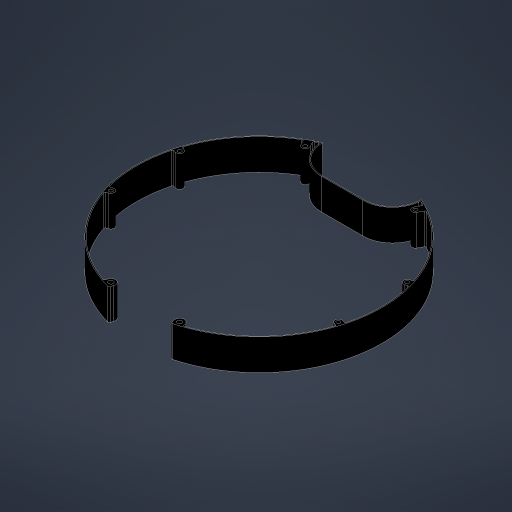
# Autodesk Inventor part: Schutz4
Saved by Autodesk Inventor 2023 (Build 270158000, 158)
## iProperties
Created: 2023-02-26
Part Number: Schutz4
Material: Generic
Document SubType Name: Modeling
Designer: Elias Braun
Density: 1 g/cm^3
Appearance: Default
Author: Elias Braun
Autodesk Inventor part; units mm, degrees
ref_plane "YZ Plane" through (0, 0, 0) normal (1, 0, 0) x (0, 1, 0)
ref_plane "XZ Plane" through (0, 0, 0) normal (0, 1, 0) x (-1, 0, 0)
ref_plane "XY Plane" through (0, 0, 0) normal (0, 0, 1) x (1, 0, 0)
sketch "Sketch1" plane through (0, 0, 0) normal (0, 1, 0) x (-1, 0, 0)
  circle A0 centre (0, 0) radius 103.75 construction
  line L0 (0, -103.75) -> (-30, -103.75) construction
  line L1 (-30, -103.75) -> (-30, -99.318) construction
  line L2 (0, -103.75) -> (0, -91.6543) construction
  line L3 (0, 0) -> (-10.2863, 0) construction
  circle A1 centre (-30, -99.318) radius 1.6
  circle A2 centre (30, -99.318) radius 1.6
  circle A3 centre (-99.318, -30) radius 1.6
  circle A4 centre (-99.318, 30) radius 1.6
  arc A5 (53.1423, -96.3114) -> (51.7739, -97.0539) centre (0, 0) ccw construction
  arc A6 (43.0581, -98.5) -> (-43.0581, -98.5) centre (0, 0) ccw
  line L4 (0, -107.5) -> (0, -98.5) construction
  line L5 (0, -98.5) -> (0, -73.5) construction
  line L6 (0, -98.5) -> (-43.0581, -98.5) construction
  line L7 (0, -98.5) -> (43.0581, -98.5) construction
  line L8 (43.0581, -98.5) -> (-43.0581, -98.5) construction
  line L9 (-18.0581, -73.5) -> (18.0581, -73.5)
  arc A7 (43.0581, -98.5) -> (18.0581, -73.5) centre (18.0581, -98.5) ccw
  arc A8 (-18.0581, -73.5) -> (-43.0581, -98.5) centre (-18.0581, -98.5) ccw
  line L10 (0, 107.5) -> (0, 97.5) construction
  line L11 (0, 97.5) -> (-22.5, 97.5) construction
  line L12 (-22.5, 97.5) -> (-22.5, 82.5) construction
  line L13 (22.5, 82.5) -> (22.5, 97.5) construction
  line L14 (22.5, 90) -> (-22.5, 90) construction
  line L15 (15, 97.5) -> (-15, 97.5)
  line L16 (-15, 82.5) -> (15, 82.5)
  arc A9 (15, 82.5) -> (15, 97.5) centre (15, 90) ccw
  arc A10 (-15, 97.5) -> (-15, 82.5) centre (-15, 90) ccw
  line L17 (22.5, 82.5) -> (17.5, 82.5) construction
  line L18 (17.5, 82.5) -> (17.5, 77.5) construction
  circle A11 centre (17.5, 77.5) radius 1.6
  circle A12 centre (-17.5, 77.5) radius 1.6
  line L19 (-58.3363, 79.5495) -> (-79.5495, 58.3363)
  arc A13 (-47.7297, 68.9429) -> (-58.3363, 79.5495) centre (-53.033, 74.2462) ccw
  arc A14 (-79.5495, 58.3363) -> (-68.9429, 47.7297) centre (-74.2462, 53.033) ccw
  line L20 (-68.9429, 47.7297) -> (-47.7297, 68.9429)
  circle A15 centre (-67.1751, 42.4264) radius 1.6
  circle A16 centre (-42.4264, 67.1751) radius 1.6
  line L21 (-97.5, 15) -> (-97.5, -15)
  arc A17 (-82.5, 15) -> (-97.5, 15) centre (-90, 15) ccw
  arc A18 (-97.5, -15) -> (-82.5, -15) centre (-90, -15) ccw
  line L22 (-82.5, -15) -> (-82.5, 15)
  circle A19 centre (-77.5, -17.5) radius 1.6
  circle A20 centre (-77.5, 17.5) radius 1.6
  line L23 (-79.5495, -58.3363) -> (-58.3363, -79.5495)
  arc A21 (-68.9429, -47.7297) -> (-79.5495, -58.3363) centre (-74.2462, -53.033) ccw
  arc A22 (-58.3363, -79.5495) -> (-47.7297, -68.9429) centre (-53.033, -74.2462) ccw
  line L24 (-47.7297, -68.9429) -> (-68.9429, -47.7297)
  circle A23 centre (-42.4264, -67.1751) radius 1.6
  circle A24 centre (-67.1751, -42.4264) radius 1.6
  line L25 (-15, -97.5) -> (15, -97.5)
  arc A25 (-15, -82.5) -> (-15, -97.5) centre (-15, -90) ccw
  arc A26 (15, -97.5) -> (15, -82.5) centre (15, -90) ccw
  line L26 (15, -82.5) -> (-15, -82.5)
  circle A27 centre (17.5, -77.5) radius 1.6
  circle A28 centre (-17.5, -77.5) radius 1.6
  line L27 (58.3363, -79.5495) -> (79.5495, -58.3363)
  arc A29 (47.7297, -68.9429) -> (58.3363, -79.5495) centre (53.033, -74.2462) ccw
  arc A30 (79.5495, -58.3363) -> (68.9429, -47.7297) centre (74.2462, -53.033) ccw
  line L28 (68.9429, -47.7297) -> (47.7297, -68.9429)
  circle A31 centre (67.1751, -42.4264) radius 1.6
  circle A32 centre (42.4264, -67.1751) radius 1.6
  line L29 (97.5, -15) -> (97.5, 15)
  arc A33 (82.5, -15) -> (97.5, -15) centre (90, -15) ccw
  arc A34 (97.5, 15) -> (82.5, 15) centre (90, 15) ccw
  line L30 (82.5, 15) -> (82.5, -15)
  circle A35 centre (77.5, 17.5) radius 1.6
  circle A36 centre (77.5, -17.5) radius 1.6
  line L31 (79.5495, 58.3363) -> (58.3363, 79.5495)
  arc A37 (68.9429, 47.7297) -> (79.5495, 58.3363) centre (74.2462, 53.033) ccw
  arc A38 (58.3363, 79.5495) -> (47.7297, 68.9429) centre (53.033, 74.2462) ccw
  line L32 (47.7297, 68.9429) -> (68.9429, 47.7297)
  circle A39 centre (42.4264, 67.1751) radius 1.6
  circle A40 centre (67.1751, 42.4264) radius 1.6
  line L33 (58.3363, -58.3363) -> (51.2652, -51.2652) construction
  line L34 (40.6586, -61.8718) -> (61.8718, -40.6586)
  arc A41 (40.6586, -61.8718) -> (44.5267, -89.5398) centre (53.033, -74.2462) ccw
  arc A42 (89.5398, -44.5267) -> (61.8718, -40.6586) centre (74.2462, -53.033) ccw
  line L35 (0, -73.5) -> (0, -66.5) construction
  arc A43 (44.5267, 89.5398) -> (40.6586, 61.8718) centre (53.033, 74.2462) ccw
  line L36 (61.8718, 40.6586) -> (40.6586, 61.8718)
  arc A44 (61.8718, 40.6586) -> (89.5398, 44.5267) centre (74.2462, 53.033) ccw
  arc A45 (-89.5398, 44.5267) -> (-61.8718, 40.6586) centre (-74.2462, 53.033) ccw
  line L37 (-40.6586, 61.8718) -> (-61.8718, 40.6586)
  arc A46 (-40.6586, 61.8718) -> (-44.5267, 89.5398) centre (-53.033, 74.2462) ccw
  arc A47 (-44.5267, -89.5398) -> (-40.6586, -61.8718) centre (-53.033, -74.2462) ccw
  line L38 (-61.8718, -40.6586) -> (-40.6586, -61.8718)
  arc A48 (-61.8718, -40.6586) -> (-89.5398, -44.5267) centre (-74.2462, -53.033) ccw
  arc A49 (89.5398, -44.5267) -> (89.5398, 44.5267) centre (0, 0) ccw
  arc A50 (-89.5398, 44.5267) -> (-89.5398, -44.5267) centre (0, 0) ccw
  line L39 (43.0581, -98.5) -> (48.0581, -98.5) construction
  line L40 (48.0581, -98.5) -> (48.0581, -88.5) construction
  circle A51 centre (48.0581, -88.5) radius 1.6
  circle A52 centre (-48.0581, -88.5) radius 1.6
  line L41 (18.0581, -66.5) -> (-18.0581, -66.5)
  arc A53 (17.5, -66.5) -> (43.0581, -59.4724) centre (19.5145, -23.8377) ccw
  arc A54 (-44.5267, -58.0038) -> (-18.0581, -66.5) centre (-19.5089, -25.5422) ccw
  circle A55 centre (30, -99.318) radius 1.6
  circle A56 centre (-30, -99.318) radius 1.6
  circle A57 centre (99.318, 30) radius 1.6
  circle A58 centre (99.318, -30) radius 1.6
  line L42 (76.014, -76.014) -> (75.4483, -75.4483) construction
  line L43 (50.8876, -93.7835) -> (51.2652, -94.4888) construction
  line L44 (51.0764, -94.1361) -> (48.0581, -88.5) construction
  line L45 (53.5045, -92.3155) -> (50.7027, -87.0837)
  line L46 (45.4135, -89.9163) -> (48.4318, -95.5524)
  arc A59 (50.7027, -87.0837) -> (45.4135, -89.9163) centre (48.0581, -88.5) ccw
  arc A60 (48.4318, -95.5524) -> (48.6295, -95.8719) centre (51.0764, -94.1361) ccw
  line L47 (102.1437, -30.8474) -> (102.9099, -31.0772) construction
  line L48 (99.318, -30) -> (102.5268, -30.9623) construction
  line L49 (98.4562, -32.8736) -> (101.2359, -33.7072)
  line L50 (103.3886, -28.0888) -> (100.1798, -27.1264)
  arc A61 (100.1798, -27.1264) -> (98.4562, -32.8736) centre (99.318, -30) ccw
  arc A62 (103.7313, -28.2147) -> (103.3886, -28.0888) centre (102.5268, -30.9623) ccw
  arc A63 (53.5045, -92.3155) -> (101.2359, -33.7072) centre (0, 0) ccw
  line L51 (102.1337, 30.8802) -> (102.8973, 31.1189) construction
  line L52 (99.318, 30) -> (102.5155, 30.9996) construction
  line L53 (100.2131, 27.1366) -> (103.4106, 28.1362)
  line L54 (101.2252, 33.7394) -> (98.4229, 32.8634)
  arc A64 (98.4229, 32.8634) -> (100.2131, 27.1366) centre (99.318, 30) ccw
  arc A65 (103.4106, 28.1362) -> (103.721, 28.2524) centre (102.5155, 30.9996) ccw
  arc A66 (102.9706, -27.9634) -> (102.9617, 27.9959) centre (0, 0) ccw
  line L55 (30.9623, 102.5268) -> (30, 99.318) construction
  line L56 (27.1309, 103.6758) -> (26.1686, 100.467)
  line L57 (33.8314, 98.1689) -> (34.6551, 100.9154)
  arc A67 (26.1686, 100.467) -> (33.8314, 98.1689) centre (30, 99.318) ccw
  arc A68 (27.2401, 103.9915) -> (27.1309, 103.6758) centre (30.9623, 102.5268) ccw
  arc A69 (101.2252, 33.7394) -> (34.6551, 100.9154) centre (0, 0) ccw
  arc A70 (44.5267, 89.5398) -> (30.2211, 95.3241) centre (0, 0) ccw
  arc A71 (-33.8314, 98.1689) -> (-26.1686, 100.467) centre (-30, 99.318) ccw
  line L58 (-33.8314, 98.1689) -> (-34.6551, 100.9154)
  line L59 (-27.1309, 103.6758) -> (-26.1686, 100.467)
  arc A72 (-27.1309, 103.6758) -> (-27.2401, 103.9915) centre (-30.9623, 102.5268) ccw
  arc A73 (26.9967, 103.2282) -> (-26.9967, 103.2282) centre (0, 0) ccw
  arc A74 (27.6048, 96.1144) -> (-27.6048, 96.1144) centre (0, 0) ccw
  arc A75 (-30.2211, 95.3241) -> (-44.5267, 89.5398) centre (0, 0) ccw
  line L60 (-101.2252, 33.7394) -> (-98.4229, 32.8634)
  arc A76 (-100.2131, 27.1366) -> (-98.4229, 32.8634) centre (-99.318, 30) ccw
  line L61 (-100.2131, 27.1366) -> (-103.4106, 28.1362)
  arc A77 (-103.721, 28.2524) -> (-103.4106, 28.1362) centre (-102.5155, 30.9996) ccw
  arc A78 (-34.6551, 100.9154) -> (-101.2252, 33.7394) centre (0, 0) ccw
  arc A79 (-102.9617, 27.9959) -> (48.2308, -95.1771) centre (0, 0) ccw
  circle A80 centre (30, 99.318) radius 2
  circle A81 centre (-30, 99.318) radius 2
  line L62 (0, -73.5) -> (0, -72.7)
  line L63 (18.0581, -72.7) -> (-18.0581, -72.7)
  arc A82 (-18.0581, -72.7) -> (-43.8294, -97.2825) centre (-18.0581, -98.5) ccw
  arc A83 (43.8294, -97.2825) -> (-43.8294, -97.2825) centre (0, 0) ccw
  arc A84 (43.8294, -97.2825) -> (18.0581, -72.7) centre (18.0581, -98.5) ccw
  circle A85 centre (-48.0581, -88.5) radius 1.6
  circle A86 centre (-99.318, -30) radius 1.6
  line L64 (-53.5045, -92.3155) -> (-50.7027, -87.0837)
  line L65 (-45.4135, -89.9163) -> (-48.4318, -95.5524)
  arc A87 (-45.4135, -89.9163) -> (-50.7027, -87.0837) centre (-48.0581, -88.5) ccw
  arc A88 (-48.6295, -95.8719) -> (-48.4318, -95.5524) centre (-51.0764, -94.1361) ccw
  line L66 (-98.4562, -32.8736) -> (-101.2359, -33.7072)
  line L67 (-103.3886, -28.0888) -> (-100.1798, -27.1264)
  arc A89 (-98.4562, -32.8736) -> (-100.1798, -27.1264) centre (-99.318, -30) ccw
  point P0 (0, 90)
  point P1 (-45.9619, 70.7107)
  point P2 (-82.5, 17.5)
  point P3 (-70.7107, -45.9619)
  point P4 (-17.5, -82.5)
  point P5 (45.9619, -70.7107)
  point P6 (82.5, -17.5)
  point P7 (70.7107, 45.9619)
  point P8 (35.7159, -76.7698)
  point P9 (49.5673, -91.3181)
  point P10 (100.9224, -30.4812)
  point P11 (100.9168, 30.4998)
  point P12 (30.4812, 100.9224)
  point P13 (-27.2401, 103.9915)
  point P14 (-103.721, 28.2524)
  point P15 (-43.8294, -97.2825)
  point P16 (-102.9706, -27.9634)
  point P17 (-48.2308, -95.1771)
  dimension "d10" = 215
  dimension "d6" = 207.5
  dimension "d7" = 30
  dimension "d8" = 3.2
  dimension "d9" = 220
  dimension "d11" = 9
  dimension "d12" = 25
  dimension "d13" = 10
  dimension "d14" = 22.5
  dimension "d15" = 15
  dimension "d16" = 45
  dimension "d17" = 5
  dimension "d18" = 5
  dimension "d19" = 3.2
  dimension "d20" = 86.1162
  dimension "d21" = 45
  dimension "d22" = 360
  dimension "d23" = 10
  dimension "d24" = 7
  dimension "d25" = 360
  dimension "d26" = 5
  dimension "d27" = 10
  dimension "d28" = 3.2
  dimension "d29" = 180
  dimension "d30" = 0.8
  dimension "d31" = 6
  dimension "d32" = 8
  dimension "d33" = 4
  dimension "d34" = 4
  dimension "d37" = 0.8
  constraints: 148 end point, 129 point on circle, 89 centre point, 30 symmetric about line, 26 point on line, 18 tangent, 12 midpoint, 10 coincident, 5 parallel, 5 vertical, 4 horizontal, 2 collinear, 2 perpendicular, 195 other
  measures "d6" diameter of A0
  measures "d7" distance of L0.start L0.end
  measures "d8" diameter of A1
  measures "d9" diameter of A5
  measures "d11" distance of L4.start L4.end
  measures "d12" distance of L4.end L5.end
  measures "d13" distance of L10.start L10.end
  measures "d14" distance of L10.end L11.end
  measures "d15" distance of L11.end L12.end
  measures "d16" distance of L12.end L13.start
  measures "d17" distance of L13.start L17.end
  measures "d18" distance of L17.end L18.end
  measures "d19" diameter of A11
  measures "d20" distance of L7.end L6.end
  measures "d21" distance of L14.start L14.end
  measures "d23" distance of L33.start L33.end
  measures "d24" distance of L5.end L35.end
  measures "d26" distance of L7.end L39.end
  measures "d27" distance of L39.end L40.end
  measures "d28" diameter of A51
  measures "d30" distance of L42.start L42.end
  measures "d31" diameter of A59
  measures "d32" diameter of A67
  measures "d33" diameter of A80
  measures "d34" diameter of A81
  measures "d37" distance of L5.end L62.end
extrude "Extrusion1" add sketch "Sketch1" along normal blind 27 contours A7 A79 L46 A60 A6 | A60 L46 A83 A63 L50 A62 A6 | A7 L9 L62 L63 A84 A41 A79 | A62 L50 A66 L53 A65 A6 | A79 A82 A47 L63 L62 L9 A8 | A8 A6 A88 L65 A79 | A65 L53 A83 A69 L56 A68 A6 | L46 A59 L45 A83 | A41 A84 | A83 L49 A61 L50 | A6 A77 L61 A79 L65 A88 | A79 L64 A87 L65 | A82 A47 | A72 L59 A83 A78 L61 A77 A6 | L53 A64 L54 A83 | A83 L57 A67 L56 | A79 L67 A89 L66 | L59 A71 L58 A83 | A83 L60 A76 L61
fillet "Fillet1" radius 1 18 edges at (-102.9706, 13.5, -27.9634) (-101.2359, 13.5, -33.7072) (-101.2252, 13.5, 33.7394) (-102.9617, 13.5, 27.9959) (-53.5045, 13.5, -92.3155) (-48.2308, 13.5, -95.1771) (53.5045, 13.5, -92.3155) (48.2308, 13.5, -95.1771) (102.9706, 13.5, -27.9634) (101.2359, 13.5, -33.7072) (102.9617, 13.5, 27.9959) (101.2252, 13.5, 33.7394) (27.2401, 13.5, 103.9915) (-27.2401, 13.5, 103.9915) (-34.6551, 13.5, 100.9154) (34.6551, 13.5, 100.9154) (-43.8294, 13.5, -97.2825) (43.8294, 13.5, -97.2825)
body "Solid1"
